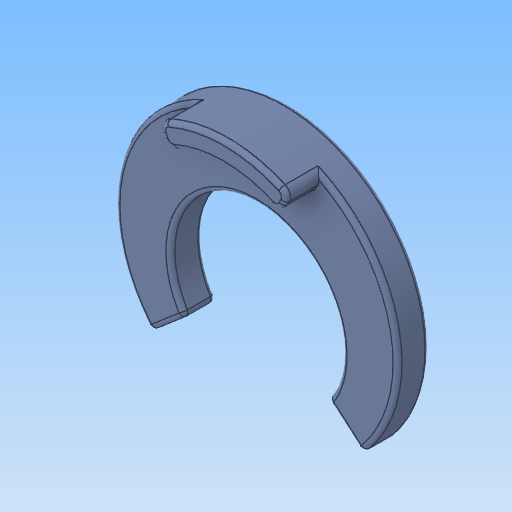
# Autodesk Inventor part: NF-Crazy   фитинг фиксатор
Saved by Autodesk Inventor 2017 (Build 210142000, 142)
## iProperties
Part Number: NF-Crazy   фитинг фиксатор
Material: Типовые
Document SubType Name: Modeling
Designer: chucha
Density: 1 g/cm^3
Appearance: Резина — синяя
Mass: 0.0956835 g
Surface Area: 2.03684 cm^2
Volume: 0.0956835 cm^3
Author: chucha
Autodesk Inventor part; units mm, degrees
ref_plane "YZ Plane" through (0, 0, 0) normal (1, 0, 0) x (0, 1, 0)
ref_plane "XZ Plane" through (0, 0, 0) normal (0, 1, 0) x (-1, 0, 0)
ref_plane "XY Plane" through (0, 0, 0) normal (0, 0, 1) x (1, 0, 0)
sketch "Эскиз1" plane through (0, 0, 0) normal (0, 0, 1) x (1, 0, 0)
  arc A0 (3.2, -2.1407) -> (-3.2, -2.1407) centre (0, 0) ccw
  arc A1 (4.7172, -3.4438) -> (-4.7172, -3.4438) centre (0, 0.7429) ccw
  line L0 (0, 0) -> (0, 13.7352) construction
  line L1 (-3.2, -2.1407) -> (-4.7172, -3.4438)
  line L2 (3.2, -2.1407) -> (4.7172, -3.4438)
  arc A2 (2.4739, 5.4381) -> (-2.4739, 5.4381) centre (0, 0.7429) ccw
  line L3 (0, 0.7429) -> (1.481, 3.5537)
  line L4 (2.4739, 5.4381) -> (2.94, 6.3229)
  line L5 (0, 0.7429) -> (-1.481, 3.5537)
  line L6 (-2.4739, 5.4381) -> (-2.94, 6.3229)
  dimension "d0" = 7.7
  dimension "d1" = 3.2
  dimension "d2" = 6.4
  dimension "d3" = 2
  dimension "d4" = 1
  constraints: 14 end point, 10 point on circle, 3 centre point, 2 coincident, 1 point on line, 1 vertical, 2 other
  measures "d0" diameter of A0
  measures "d2" distance of L1.start L2.start
  measures "d3" distance of L2.start L2.end
  measures "d4" radial gap between concentric circles of A1 A2
extrude "Выдавливание1" add sketch "Эскиз1" along normal blind 1.43 contours A0 L1 A1 L6 A2 L4 L2
extrude "Выдавливание2" add sketch "Эскиз1" along normal blind 2.9 contours L4 A2 L6 A1
fillet "Сопряжение1" radius 0.4 4 edges at (2.4739, 5.4381, 2.165) (2.94, 6.3229, 2.165) (-2.94, 6.3229, 2.165) (-2.4739, 5.4381, 2.165)
fillet "Сопряжение2" radius 0.2 15 edges at (2.7493, 6.4193, 1.43) (6.2052, 1.872, 1.43) (-2.7493, 6.4193, 1.43) (-6.2052, 1.872, 1.43) (-3.9586, -2.7922, 1.43) (0, 3.85, 1.43) (0, 7.05, 0) (-3.9586, -2.7922, 0) (0, 3.85, 0) (3.9586, -2.7922, 0) (4.7172, -3.4438, 0.715) (3.2, -2.1407, 0.715) (-3.2, -2.1407, 0.715) (3.9586, -2.7922, 1.43) (-4.7172, -3.4438, 0.715)
fillet "Сопряжение3" radius 0.2 8 edges at (2.4316, 5.5884, 2.9) (2.7005, 5.8683, 2.9) (2.7712, 6.2747, 2.9) (0, 7.05, 2.9) (-2.7712, 6.2747, 2.9) (-2.7005, 5.8683, 2.9) (-2.4316, 5.5884, 2.9) (0, 6.05, 2.9)
